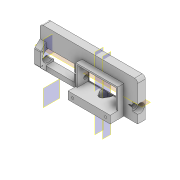
# Autodesk Inventor part: 10_Wellplate_base_v1
Saved by Autodesk Inventor 2022 (Build 260153000, 153)
## iProperties
Created: 2022-04-18
Part Number: 10_Wellplate_base_v1
Material: Generic
Document SubType Name: Modeling
Designer: Prakash Lab
Density: 1 g/cm^3
Appearance: Default
Author: Prakash Lab
Autodesk Inventor part; units mm, degrees
ref_plane "YZ Plane" through (0, 0, 0) normal (1, 0, 0) x (0, 1, 0)
ref_plane "XZ Plane" through (0, 0, 0) normal (0, 1, 0) x (-1, 0, 0)
ref_plane "XY Plane" through (0, 0, 0) normal (0, 0, 1) x (1, 0, 0)
sketch "Sketch1" plane through (0, 0, 0) normal (0, 0, 1) x (1, 0, 0)
  line L0 (63.9, -42.75) -> (-63.9, -42.75)
  line L1 (-63.9, -42.75) -> (-63.9, 42.75)
  line L2 (-63.9, 42.75) -> (63.9, 42.75)
  line L3 (63.9, 42.75) -> (63.9, -42.75)
  line L4 (63.9, -42.75) -> (-63.9, 42.75) construction
  line L5 (-63.9, -42.75) -> (63.9, 42.75) construction
  point P0 (0, 0)
  dimension "d0" = 127.8
  dimension "d1" = 85.5
  constraints: 12 end point, 2 midpoint, 2 parallel, 1 horizontal, 1 perpendicular
  measures "d0" distance of L0.start L0.end
  measures "d1" distance of L0.end L1.end
extrude "Extrusion1" add sketch "Sketch1" along normal blind 10
fillet "Fillet1" radius 4 4 edges at (63.9, 42.75, 5) (-63.9, 42.75, 5) (-63.9, -42.75, 5) (63.9, -42.75, 5)
sketch "Sketch2" plane through (0, 0, 10) normal (0, 0, 1) x (1, 0, 0)
  arc A0 (59.9, -42.75) -> (63.9, -38.75) centre (59.9, -38.75) ccw projected
  line L0 (63.9, -38.75) -> (63.9, 38.75) projected
  arc A1 (63.9, 38.75) -> (59.9, 42.75) centre (59.9, 38.75) ccw projected
  line L1 (59.9, 42.75) -> (-59.9, 42.75) projected
  arc A2 (-59.9, 42.75) -> (-63.9, 38.75) centre (-59.9, 38.75) ccw projected
  line L2 (-63.9, 38.75) -> (-63.9, -38.75) projected
  arc A3 (-63.9, -38.75) -> (-59.9, -42.75) centre (-59.9, -38.75) ccw projected
  line L3 (-59.9, -42.75) -> (59.9, -42.75) projected
  line L4 (43.9, 2.75) -> (-7.1, 2.75)
  line L5 (-7.1, 2.75) -> (-7.1, 27.75)
  line L6 (-7.1, 27.75) -> (43.9, 27.75)
  line L7 (43.9, 27.75) -> (43.9, 2.75)
  line L8 (43.9, 2.75) -> (-7.1, 27.75) construction
  line L9 (-7.1, 2.75) -> (43.9, 27.75) construction
  point P0 (0, 0)
  point P1 (18.4, 15.25)
  dimension "d5" = 51
  dimension "d6" = 25
  dimension "d7" = 20
  dimension "d8" = 15
  constraints: 12 end point, 2 midpoint, 2 parallel, 1 horizontal, 1 perpendicular
  measures "d5" distance of L5.end L6.end
  measures "d6" distance of L4.end L5.end
  measures "d7" distance between parallel lines of L0 L7
  measures "d8" distance between parallel lines of L6 L1
extrude "Extrusion2" cut sketch "Sketch2" against normal blind 6 contours L4 L5 L6 L7
sketch "Sketch3" plane through (0, 0, 4) normal (0, 0, 1) x (1, 0, 0)
  line L0 (-7.1, 27.75) -> (43.9, 27.75) projected
  line L1 (-7.1, 2.75) -> (-7.1, 27.75) projected
  line L2 (43.9, 2.75) -> (-7.1, 2.75) projected
  line L3 (43.9, 27.75) -> (43.9, 2.75) projected
  line L4 (42.4, 26.25) -> (-5.6, 26.25)
  line L5 (-5.6, 26.25) -> (-5.6, 4.25)
  line L6 (-5.6, 4.25) -> (42.4, 4.25)
  line L7 (42.4, 4.25) -> (42.4, 26.25)
  point P0 (0, 0)
  dimension "d11" = 1.5
  constraints: 8 end point, 3 other
  measures "d11" distance between parallel lines of L0 L4
extrude "Extrusion3" cut sketch "Sketch3" against normal through all contours L7 L6 L5 L4
ref_plane "Work Plane1" through (18.4, 2.75, 10) normal (-1, 0, 0) x (0, 0, 1)
ref_plane "Work Plane2" through (-7.1, 15.25, 10) normal (0, 1, 0) x (1, 0, 0)
chamfer "Chamfer1" distance 4 angle 45 4 edges at (18.4, 4.25, 0) (42.4, 15.25, 0) (18.4, 26.25, 0) (-5.6, 15.25, 0)
sketch "Sketch4" plane through (0, 0, 10) normal (0, 0, 1) x (1, 0, 0)
  line L0 (-7.1, 2.75) -> (-7.1, 27.75) projected
  line L1 (-7.1, 27.75) -> (43.9, 27.75) projected
  line L2 (43.9, 27.75) -> (43.9, 2.75) projected
  line L3 (43.9, 2.75) -> (-7.1, 2.75) projected
  arc A0 (59.9, -42.75) -> (63.9, -38.75) centre (59.9, -38.75) ccw projected
  line L4 (63.9, -38.75) -> (63.9, 38.75) projected
  arc A1 (63.9, 38.75) -> (59.9, 42.75) centre (59.9, 38.75) ccw projected
  line L5 (59.9, 42.75) -> (-59.9, 42.75) projected
  arc A2 (-59.9, 42.75) -> (-63.9, 38.75) centre (-59.9, 38.75) ccw projected
  line L6 (-63.9, 38.75) -> (-63.9, -38.75) projected
  arc A3 (-63.9, -38.75) -> (-59.9, -42.75) centre (-59.9, -38.75) ccw projected
  line L7 (-59.9, -42.75) -> (59.9, -42.75) projected
  line L8 (-7.1, 2.75) -> (43.9, 2.75)
  line L9 (43.9, 2.75) -> (43.9, -7.25)
  line L10 (43.9, -7.25) -> (-7.1, -7.25)
  line L11 (-7.1, -7.25) -> (-7.1, 2.75)
  line L12 (-7.1, 27.75) -> (43.9, 27.75) projected
  line L13 (-7.1, 27.75) -> (-9.1, 27.75)
  line L14 (-9.1, 27.75) -> (-9.1, -7.25)
  line L15 (-9.1, -7.25) -> (-7.1, -7.25)
  line L16 (-7.1, -7.25) -> (-7.1, 27.75)
  line L17 (43.9, 27.75) -> (45.9, 27.75)
  line L18 (45.9, 27.75) -> (45.9, -7.25)
  line L19 (45.9, -7.25) -> (43.9, -7.25)
  line L20 (43.9, -7.25) -> (43.9, 27.75)
  line L21 (45.9, 27.75) -> (-9.1, 27.75)
  line L22 (-9.1, 27.75) -> (-9.1, 29.75)
  line L23 (-9.1, 29.75) -> (45.9, 29.75)
  line L24 (45.9, 29.75) -> (45.9, 27.75)
  point P0 (0, 0)
  dimension "d17" = 10
  dimension "d52" = 2
  dimension "d53" = 2
  dimension "d54" = 2
  constraints: 32 end point, 8 parallel, 4 horizontal, 4 perpendicular, 2 point on line
  measures "d17" distance of L8.end L9.end
  measures "d52" distance of L15.end L14.end
  measures "d53" distance of L18.end L19.end
  measures "d54" distance of L21.end L22.end
extrude "Extrusion4" add sketch "Sketch4" along normal blind 8 contours L11 L15 L14 L13 L0 | L3 L9 L10 L11 | L13 L22 L23 L24 L17 L1 | L2 L17 L18 L19 L9
sketch "Sketch5" plane through (-7.1, 2.75, 4) normal (0, 1, 0) x (1, 0, 0)
  line L0 (22.0359, -8.925) -> (18.745, -3.225)
  line L1 (22.2091, 2.775) -> (28.7909, 2.775)
  line L2 (32.255, -3.225) -> (28.9641, -8.925)
  line L3 (53.5, 4) -> (-2.5, 4) projected
  circle A0 centre (25.5, -3.125) radius 0.95
  arc A1 (22.0359, -8.925) -> (28.9641, -8.925) centre (25.5, -6.925) ccw
  arc A2 (22.2091, 2.775) -> (18.745, -3.225) centre (22.2091, -1.225) ccw
  arc A3 (32.255, -3.225) -> (28.7909, 2.775) centre (28.7909, -1.225) ccw
  circle A4 centre (25.5, -3.125) radius 5.9
  circle A5 centre (25.5, -3.125) radius 6 projected
  point P0 (7.1, 4)
  point P1 (25.5, -14.925)
  point P2 (15.2809, 2.775)
  point P3 (35.7191, 2.775)
  dimension "d20" = 1.9
  dimension "d21" = 4
  dimension "d103" = 11.8
  constraints: 7 tangent, 6 end point, 6 point on circle, 6 point on line, 5 centre point, 3 coincident, 2 equal radius, 1 parallel, 7 other
  measures "d20" diameter of A0
  measures "d21" radius of A1
  measures "d103" diameter of A4
extrude "Extrusion5" cut sketch "Sketch5" against normal up to surface (10 mm away) contours L0 A5 L2 A1 | L0 A4 L2 A5 | L0 A5 L1 A4 | A4 | L0 A2 L1 A5 | L1 A5 L2 A4 | A5 L1 A3 L2 | A0
sketch "Sketch6" plane through (18.4, -7.25, 11.125) normal (0, -1, 0) x (1, 0, 0)
  circle A0 centre (0, -4) radius 7 projected
  circle A1 centre (0, -4) radius 10
  point P0 (-18.4, -11.125)
  dimension "d27" = 20
  constraints: 1 centre point, 1 coincident
  measures "d27" diameter of A1
extrude "Extrusion6" cut sketch "Sketch6" along normal blind 18 contours A0 | A1
ref_plane "Work Plane3" through (8.4, 2.75, 10) normal (-1, 0, 0) x (0, 0, 1)
sketch "Sketch12" plane through (63.9, -38.75, 0) normal (1, 0, 0) x (0, 0, -1)
  circle A0 centre (-7.125, 48) radius 4.2 construction
  circle A1 centre (-7.125, 48) radius 3.5
  point P0 (0, 38.75)
  dimension "d100" = 7
  constraints: 1 centre point
  measures "d100" diameter of A1
extrude "Extrusion12" cut sketch "Sketch12" against normal blind 30 draft -3
sketch "Sketch13" plane through (63.9, -38.75, 0) normal (1, 0, 0) x (0, 0, -1)
  arc A0 (-10, 44.9382) -> (-10, 51.0618) centre (-7.125, 48) ccw projected
  circle A1 centre (-7.125, 48) radius 6
  point P0 (0, 38.75)
  dimension "d63" = 12
  constraints: 1 centre point, 1 coincident
  measures "d63" diameter of A1
extrude "Extrusion13" cut sketch "Sketch13" against normal blind 7
mirror "Mirror1" about plane through (18.4, 2.75, 10) normal (-1, 0, 0) of "Extrusion12", "Extrusion13"
ref_plane "Work Plane4" through (-47.9, 27.75, 11) normal (-1, 0, 0) x (0, 0, 1)
ref_plane "Work Plane5" through (-39.7, 19.25, 21) normal (0, 0, 1) x (1, 0, 0)
sketch "Sketch22" plane through (0, 0, 18) normal (0, 0, 1) x (1, 0, 0)
  line L0 (-7.1, 2.75) -> (-7.1, 27.75) projected
  line L1 (-7.1, 27.75) -> (43.9, 27.75) projected
  line L2 (43.9, 27.75) -> (43.9, 2.75) projected
  line L3 (43.9, 2.75) -> (-7.1, 2.75) projected
  line L4 (-9.1, -7.25) -> (45.9, -7.25) projected
  line L5 (45.9, -7.25) -> (45.9, 29.75) projected
  line L6 (45.9, 29.75) -> (-9.1, 29.75) projected
  line L7 (-9.1, 29.75) -> (-9.1, -7.25) projected
  line L8 (45.9, -7.25) -> (45.9, 29.75) projected
  line L9 (45.9, 2.75) -> (-9.1, 2.75)
  point P0 (0, 0)
  point P1 (43.9, 2.75)
  constraints: 2 end point, 2 point on line, 1 perpendicular
extrude "Extrusion21" add sketch "Sketch22" along normal blind 10 contours L3 L9 L5 L4 L7
sketch "Sketch23" plane through (0, 0, 28) normal (0, 0, 1) x (1, 0, 0)
  line L0 (45.9, -7.25) -> (45.9, 2.75) projected
  line L1 (45.9, 2.75) -> (-9.1, 2.75) projected
  line L2 (-9.1, 2.75) -> (-9.1, -7.25) projected
  line L3 (-9.1, -7.25) -> (45.9, -7.25) projected
  circle A0 centre (39.9, -2.25) radius 1.4
  circle A1 centre (-3.1, -2.25) radius 1.4
  point P0 (0, 0)
  dimension "d105" = 2.8
  dimension "d106" = 2.8
  dimension "d107" = 6
  dimension "d108" = 6
  constraints: 2 centre point
  measures "d105" diameter of A0
  measures "d106" diameter of A1
  measures "d107" distance from line of A0.centre L0
  measures "d108" distance from line of A1.centre L2
extrude "Extrusion22" cut sketch "Sketch23" against normal through all contours A0 | A1
ref_plane "Arbeitsebene7" through (-58.9, -38.75, 0) normal (-1, 0, 0) x (0, 0, 1)
sketch "Skizze28" plane through (-58.9, -38.75, 0) normal (-1, 0, 0) x (0, 0, 1)
  line L0 (17.125, 56.5) -> (17.125, 39.5) projected
  arc A0 (17.125, 56.5) -> (15.625, 58) centre (15.625, 56.5) ccw projected
  line L1 (-1.375, 58) -> (15.625, 58) projected
  arc A1 (-1.375, 58) -> (-2.875, 56.5) centre (-1.375, 56.5) ccw projected
  line L2 (-2.875, 39.5) -> (-2.875, 56.5) projected
  arc A2 (-2.875, 39.5) -> (-1.375, 38) centre (-1.375, 39.5) ccw projected
  line L3 (15.625, 38) -> (-1.375, 38) projected
  arc A3 (15.625, 38) -> (17.125, 39.5) centre (15.625, 39.5) ccw projected
  circle A4 centre (15.125, 56) radius 0.7835 projected
  circle A5 centre (15.125, 40) radius 0.7835 projected
  circle A6 centre (-0.875, 56) radius 0.7835 projected
  circle A7 centre (-0.875, 40) radius 0.7835 projected
  circle A8 centre (7.125, 48) radius 7.5 projected
  arc A9 (17.625, 56.5) -> (15.625, 58.5) centre (15.625, 56.5) ccw
  line L4 (17.625, 56.5) -> (17.625, 39.5)
  arc A10 (15.625, 37.5) -> (17.625, 39.5) centre (15.625, 39.5) ccw
  line L5 (15.625, 37.5) -> (-1.375, 37.5)
  arc A11 (-3.375, 39.5) -> (-1.375, 37.5) centre (-1.375, 39.5) ccw
  line L6 (-3.375, 39.5) -> (-3.375, 56.5)
  arc A12 (-1.375, 58.5) -> (-3.375, 56.5) centre (-1.375, 56.5) ccw
  line L7 (-1.375, 58.5) -> (15.625, 58.5)
  point P0 (0, 38.75)
  dimension "d142" = 0.5
  constraints: 8 end point, 8 point on circle, 4 centre point, 7 other
  measures "d142" distance between parallel lines of L1 L7
extrude "Extrusion27" cut sketch "Skizze28" against normal blind 40 contours L0 A3 L3 A2 L2 A1 L1 A0 | A4 | A5 | A6 | A7 | A8 | L4 A10 L5 A11 L6 A12 L7 A9
sketch "Skizze29" plane through (-63.9, -38.75, 0) normal (-1, 0, 0) x (0, 0, 1)
  line L0 (17.125, 56.5) -> (17.125, 39.5) projected
  arc A0 (17.125, 56.5) -> (15.625, 58) centre (15.625, 56.5) ccw projected
  line L1 (-1.375, 58) -> (15.625, 58) projected
  arc A1 (-1.375, 58) -> (-2.875, 56.5) centre (-1.375, 56.5) ccw projected
  line L2 (-2.875, 39.5) -> (-2.875, 56.5) projected
  arc A2 (-2.875, 39.5) -> (-1.375, 38) centre (-1.375, 39.5) ccw projected
  line L3 (15.625, 38) -> (-1.375, 38) projected
  arc A3 (15.625, 38) -> (17.125, 39.5) centre (15.625, 39.5) ccw projected
  circle A4 centre (15.125, 56) radius 0.7835 projected
  circle A5 centre (15.125, 40) radius 0.7835 projected
  circle A6 centre (-0.875, 56) radius 0.7835 projected
  circle A7 centre (-0.875, 40) radius 0.7835 projected
  circle A8 centre (7.125, 48) radius 7.5 projected
  line L4 (0, 77.5) -> (0, 0) projected
  line L5 (10, 77.5) -> (10, 0) projected
  line L6 (10, 0) -> (10, 42.7337) projected
  line L7 (10, 31.7537) -> (16.6857, 38.4393)
  line L8 (16.6857, 57.5607) -> (10, 64.2463)
  line L9 (10, 68.5) -> (10, 31.5) projected
  point P0 (0, 38.75)
  point P1 (0, 58)
  point P2 (0, 38)
  point P3 (10, 11.9077)
  point P4 (10, 38)
  point P5 (10, 58)
  point P6 (10, 10.3787)
  dimension "d151" = 45
  dimension "d152" = 45
  constraints: 4 end point, 2 point on circle, 2 point on line
  measures "d151" angle of L1 L8
  measures "d152" angle of L3 L7
extrude "Extrusion28" add sketch "Skizze29" against normal blind 8 contours L0 A3 L3 L5 A8 L1 A0 | A0 L1 L5 L8 | L7 L5 L3 A3 | L5 A8 L4 L1 | L3 L4 A8 L5 | L5 A8 L4 | A8 L5
sketch "Skizze30" plane through (-55.9, -38.75, 0) normal (1, 0, 0) x (0, 0, -1)
  circle A0 centre (-7.125, 48) radius 7.3 projected
  circle A1 centre (-7.125, 48) radius 7.8
  point P0 (0, 38.75)
  dimension "d147" = 0.5
  constraints: 1 centre point
  measures "d147" radial gap between concentric circles of A0 A1
extrude "Extrusion29" cut sketch "Skizze30" against normal up to surface (8 mm away) contours A0 | A1
fillet "Rundung6" radius 2 2 edges at (-59.9, 6.076, 0) (-59.9, 12.424, 0)
sketch "Skizze32" plane through (-63.9, -38.75, 0) normal (-1, 0, 0) x (0, 0, 1)
  circle A0 centre (5.1474, 11) radius 6.7945 projected
  point P0 (0, 38.75)
ref_plane "Arbeitsebene8" through (-41.36, -34.2905, -1.3931) normal (1, 0, 0) x (0, 1, 0)
extrude "Extrusion30" cut sketch "Skizze32" against normal up to surface (22.54 mm away)
sketch "Skizze33" plane through (-41.36, -32.5058, 10) normal (-1, 0, 0) x (0, 0, 1)
  arc A0 (-5.8686, 8.6246) -> (-3.8366, 8.6246) centre (-4.8526, 4.7558) ccw projected
  circle A1 centre (-4.8526, 4.7558) radius 3.5
  line L0 (-4.8526, 8.2558) -> (5.2065, 8.2558)
  line L1 (5.2065, 8.2558) -> (5.2065, 1.2558)
  line L2 (5.2065, 1.2558) -> (-4.8526, 1.2558)
  line L3 (-4.8526, 1.2558) -> (-4.8526, 8.2558)
  point P0 (-10, 32.5058)
  point P1 (-4.8526, 1.2558)
  dimension "d155" = 7
  constraints: 8 end point, 2 parallel, 1 coincident, 1 horizontal, 1 perpendicular, 3 other
extrude "Extrusion31" cut sketch "Skizze33" against normal blind 3
sketch "Skizze34" plane through (-38.36, -32.5058, 10) normal (-1, 0, 0) x (0, 0, 1)
  circle A0 centre (-4.8526, 4.7558) radius 6.5405 projected
  circle A1 centre (-4.8526, 4.7558) radius 8.5
  line L0 (-4.8526, 13.2558) -> (8.37, 13.2558)
  line L1 (8.37, 13.2558) -> (8.37, -3.7442)
  line L2 (8.37, -3.7442) -> (-4.8526, -3.7442)
  line L3 (-4.8526, -3.7442) -> (-4.8526, 13.2558)
  point P0 (-10, 32.5058)
  point P1 (-4.8526, -3.7442)
  dimension "d160" = 17
  constraints: 8 end point, 2 parallel, 1 coincident, 1 horizontal, 1 perpendicular, 3 other
extrude "Extrusion32" cut sketch "Skizze34" against normal blind 30
sketch "Skizze35" plane through (-38.36, -32.5058, 10) normal (1, 0, 0) x (0, 0, -1)
  line L0 (10, 11.52) -> (10, -2.0084) projected
  arc A0 (10, 11.52) -> (4.8526, 13.2558) centre (4.8526, 4.7558) ccw projected
  line L1 (0, 13.2558) -> (4.8526, 13.2558) projected
  line L2 (0, 8.2558) -> (0, 13.2558) projected
  line L3 (4.8526, 8.2558) -> (0, 8.2558) projected
  arc A1 (4.8526, 1.2558) -> (4.8526, 8.2558) centre (4.8526, 4.7558) ccw projected
  line L4 (0, 1.2558) -> (4.8526, 1.2558) projected
  line L5 (0, -3.7442) -> (0, 1.2558) projected
  line L6 (4.8526, -3.7442) -> (0, -3.7442) projected
  arc A2 (4.8526, -3.7442) -> (10, -2.0084) centre (4.8526, 4.7558) ccw projected
  circle A3 centre (4.8526, 4.7558) radius 6 projected
  line L7 (4.8526, 10.7558) -> (0, 10.7558)
  line L8 (4.8526, -1.2442) -> (0, -1.2442)
  line L9 (0, -3.7442) -> (0, 1.2558) projected
  point P0 (10, 32.5058)
  point P1 (10, 1.6729)
  point P2 (0, -1.2442)
  point P3 (10, 7.8387)
  constraints: 4 end point, 2 midpoint, 2 point on circle
extrude "Extrusion33" add sketch "Skizze35" along normal blind 15 contours L0 A3 L7 L2 L1 A0 | L0 A2 L6 L5 L8 A3
sketch "Skizze36" plane through (0, 0, 10) normal (0, 0, 1) x (1, 0, 0)
  line L0 (20.65, -24.75) -> (15.25, -24.75) projected
  line L1 (15.25, -24.75) -> (15.25, -31.55) projected
  line L2 (20.65, -31.55) -> (15.25, -31.55) projected
  line L3 (20.65, -31.55) -> (20.65, -24.75) projected
  line L4 (14.75, -32.05) -> (14.75, -24.25)
  line L5 (14.75, -24.25) -> (21.15, -24.25)
  line L6 (21.15, -24.25) -> (21.15, -32.05)
  line L7 (21.15, -32.05) -> (14.75, -32.05)
  point P0 (0, 0)
  dimension "d163" = 0.5
  constraints: 8 end point, 3 other
  measures "d163" distance between parallel lines of L1 L4
ref_plane "Arbeitsebene9" through (15.25, -31.55, 0.625) normal (0, 0, -1) x (0, 1, 0)
extrude "Extrusion34" cut sketch "Skizze36" against normal up to surface (9.375 mm away) contours L3 L2 L1 L0 | L4 L5 L6 L7
sketch "Skizze37" plane through (-8.36, -32.5058, 10) normal (-1, 0, 0) x (0, 0, 1)
  circle A0 centre (-4.8526, 4.7558) radius 6.5405 projected
  circle A1 centre (-4.8526, 4.7558) radius 4
  line L0 (-4.8526, 0.7558) -> (5.4732, 0.7558)
  line L1 (5.4732, 0.7558) -> (5.4732, 8.7558)
  line L2 (5.4732, 8.7558) -> (-4.8526, 8.7558)
  line L3 (-4.8526, 8.7558) -> (-4.8526, 0.7558)
  point P0 (-10, 32.5058)
  point P1 (-4.8526, 8.7558)
  dimension "d166" = 8
  constraints: 8 end point, 2 parallel, 1 coincident, 1 horizontal, 1 perpendicular, 3 other
extrude "Extrusion35" cut sketch "Skizze37" against normal up to surface (23.11 mm away) contours A0 L0 A1 L2 | A0 L2 L1 L0 | L3 A1 | A1 L3 picked at (0.7888, 4.2814)
sketch "Skizze38" plane through (0, 0, 10) normal (0, 0, 1) x (1, 0, 0)
  line L0 (-8.36, -23.75) -> (8.8222, -23.75) projected
  line L1 (8.8222, -23.75) -> (8.8222, -7.25) projected
  line L2 (8.8222, -7.25) -> (-9.1, -7.25) projected
  line L3 (-9.1, -7.25) -> (-9.1, 29.75) projected
  line L4 (-9.1, 29.75) -> (45.9, 29.75) projected
  line L5 (45.9, 29.75) -> (45.9, -7.25) projected
  line L6 (45.9, -7.25) -> (27.9778, -7.25) projected
  line L7 (27.9778, -7.25) -> (27.9778, -25.25) projected
  line L8 (27.9778, -25.25) -> (21.15, -25.25) projected
  line L9 (21.15, -25.25) -> (21.15, -32.05) projected
  line L10 (21.15, -32.05) -> (14.75, -32.05) projected
  line L11 (14.75, -32.05) -> (14.75, -31.75) projected
  line L12 (14.75, -31.75) -> (-8.36, -31.75) projected
  line L13 (-8.36, -31.75) -> (-8.36, -36.25) projected
  line L14 (-8.36, -36.25) -> (-23.36, -36.25) projected
  line L15 (-23.36, -33.75) -> (-23.36, -36.25) projected
  line L16 (-38.36, -33.75) -> (-23.36, -33.75) projected
  line L17 (-38.36, -33.75) -> (-38.36, -31.25) projected
  line L18 (-38.36, -31.25) -> (-41.36, -31.25) projected
  line L19 (-41.36, -31.25) -> (-41.36, -32.5058) projected
  line L20 (-41.36, -32.5058) -> (-63.9, -32.5058) projected
  line L21 (-63.9, -32.5058) -> (-63.9, -38.75) projected
  arc A0 (-63.9, -38.75) -> (-59.9, -42.75) centre (-59.9, -38.75) ccw projected
  line L22 (-59.9, -42.75) -> (59.9, -42.75) projected
  arc A1 (59.9, -42.75) -> (63.9, -38.75) centre (59.9, -38.75) ccw projected
  line L23 (63.9, -38.75) -> (63.9, 3.9837) projected
  line L24 (63.9, 3.9837) -> (56.9, 3.9837) projected
  line L25 (56.9, 3.9837) -> (56.9, 8.0046) projected
  line L26 (56.9, 10.4954) -> (56.9, 14.5163) projected
  line L27 (56.9, 14.5163) -> (63.9, 14.5163) projected
  line L28 (63.9, 14.5163) -> (63.9, 38.75) projected
  arc A2 (63.9, 38.75) -> (59.9, 42.75) centre (59.9, 38.75) ccw projected
  line L29 (59.9, 42.75) -> (-59.9, 42.75) projected
  arc A3 (-59.9, 42.75) -> (-63.9, 38.75) centre (-59.9, 38.75) ccw projected
  line L30 (-63.9, 38.75) -> (-63.9, 25.4963) projected
  line L31 (-63.9, 25.4963) -> (-55.9, 25.4963) projected
  line L32 (-55.9, 25.4963) -> (-55.9, 19.75) projected
  line L33 (-55.9, 19.75) -> (-18.9, 19.75) projected
  line L34 (-18.9, 19.75) -> (-18.9, 10.3274) projected
  line L35 (-18.9, 8.1726) -> (-18.9, -1.25) projected
  line L36 (-18.9, -1.25) -> (-55.9, -1.25) projected
  line L37 (-55.9, -1.25) -> (-55.9, -6.9963) projected
  line L38 (-55.9, -6.9963) -> (-63.9, -6.9963) projected
  line L39 (-63.9, -6.9963) -> (-63.9, -22.9942) projected
  line L40 (-63.9, -22.9942) -> (-41.36, -22.9942) projected
  line L41 (-41.36, -22.9942) -> (-41.36, -24.25) projected
  line L42 (-41.36, -24.25) -> (-38.36, -24.25) projected
  line L43 (-38.36, -24.25) -> (-38.36, -21.75) projected
  line L44 (-38.36, -21.75) -> (-23.36, -21.75) projected
  line L45 (-23.36, -19.25) -> (-23.36, -21.75) projected
  line L46 (-23.36, -19.25) -> (-8.36, -19.25) projected
  line L47 (-8.36, -19.25) -> (-8.36, -23.75) projected
  point P0 (0, 0)
  point P1 (-42.2276, -36.25)
  point P2 (-42.2276, -19.25)
  point P3 (-27.8589, -14.9953)
  point P4 (-27.8589, -39.949)
  point P5 (17.95, -36.25)
  point P6 (27.4914, -28.65)
  point P7 (5.4922, -12.0867)
  point P8 (32.285, -12.0867)
  constraints: 2 vertical alignment
hole "Bohrung2" at (-42.2276, -36.25, 10) at (-42.2276, -19.25, 10) at (-27.8589, -14.9953, 10) at (-27.8589, -39.949, 10) at (17.95, -36.25, 10) at (27.4914, -28.65, 10) at (5.4922, -12.0867, 10) at (32.285, -12.0867, 10) direction (0, 0, -1) diameter 2.8 end through all
sketch "Skizze39" plane through (0, 0, 10) normal (0, 0, 1) x (1, 0, 0)
  circle A0 centre (5.4922, -12.0867) radius 1.4 projected
  circle A1 centre (17.95, -36.25) radius 1.4 projected
  circle A2 centre (-27.8589, -14.9953) radius 1.4 projected
  circle A3 centre (-42.2276, -36.25) radius 1.4 projected
  circle A4 centre (-42.2276, -19.25) radius 1.4 projected
  circle A5 centre (-27.8589, -39.949) radius 1.4 projected
  circle A6 centre (27.4914, -28.65) radius 1.4 projected
  circle A7 centre (32.285, -12.0867) radius 1.4 projected
  line L0 (-8.36, -23.75) -> (8.8222, -23.75) projected
  line L1 (8.8222, -23.75) -> (8.8222, -7.25) projected
  line L2 (8.8222, -7.25) -> (-9.1, -7.25) projected
  line L3 (-9.1, -7.25) -> (-9.1, 29.75) projected
  line L4 (-9.1, 29.75) -> (45.9, 29.75) projected
  line L5 (45.9, 29.75) -> (45.9, -7.25) projected
  line L6 (45.9, -7.25) -> (27.9778, -7.25) projected
  line L7 (27.9778, -7.25) -> (27.9778, -25.25) projected
  line L8 (27.9778, -25.25) -> (21.15, -25.25) projected
  line L9 (21.15, -25.25) -> (21.15, -32.05) projected
  line L10 (21.15, -32.05) -> (14.75, -32.05) projected
  line L11 (14.75, -32.05) -> (14.75, -31.75) projected
  line L12 (14.75, -31.75) -> (-8.36, -31.75) projected
  line L13 (-8.36, -31.75) -> (-8.36, -36.25) projected
  line L14 (-8.36, -36.25) -> (-23.36, -36.25) projected
  line L15 (-23.36, -33.75) -> (-23.36, -36.25) projected
  line L16 (-38.36, -33.75) -> (-23.36, -33.75) projected
  line L17 (-38.36, -33.75) -> (-38.36, -31.25) projected
  line L18 (-38.36, -31.25) -> (-41.36, -31.25) projected
  line L19 (-41.36, -31.25) -> (-41.36, -32.5058) projected
  line L20 (-41.36, -32.5058) -> (-63.9, -32.5058) projected
  line L21 (-63.9, -32.5058) -> (-63.9, -38.75) projected
  arc A8 (-63.9, -38.75) -> (-59.9, -42.75) centre (-59.9, -38.75) ccw projected
  line L22 (-59.9, -42.75) -> (59.9, -42.75) projected
  arc A9 (59.9, -42.75) -> (63.9, -38.75) centre (59.9, -38.75) ccw projected
  line L23 (63.9, -38.75) -> (63.9, 3.9837) projected
  line L24 (63.9, 3.9837) -> (56.9, 3.9837) projected
  line L25 (56.9, 3.9837) -> (56.9, 8.0046) projected
  line L26 (56.9, 10.4954) -> (56.9, 14.5163) projected
  line L27 (56.9, 14.5163) -> (63.9, 14.5163) projected
  line L28 (63.9, 14.5163) -> (63.9, 38.75) projected
  arc A10 (63.9, 38.75) -> (59.9, 42.75) centre (59.9, 38.75) ccw projected
  line L29 (59.9, 42.75) -> (-59.9, 42.75) projected
  arc A11 (-59.9, 42.75) -> (-63.9, 38.75) centre (-59.9, 38.75) ccw projected
  line L30 (-63.9, 38.75) -> (-63.9, 25.4963) projected
  line L31 (-63.9, 25.4963) -> (-55.9, 25.4963) projected
  line L32 (-55.9, 25.4963) -> (-55.9, 19.75) projected
  line L33 (-55.9, 19.75) -> (-18.9, 19.75) projected
  line L34 (-18.9, 19.75) -> (-18.9, 10.3274) projected
  line L35 (-18.9, 8.1726) -> (-18.9, -1.25) projected
  line L36 (-18.9, -1.25) -> (-55.9, -1.25) projected
  line L37 (-55.9, -1.25) -> (-55.9, -6.9963) projected
  line L38 (-55.9, -6.9963) -> (-63.9, -6.9963) projected
  line L39 (-63.9, -6.9963) -> (-63.9, -22.9942) projected
  line L40 (-63.9, -22.9942) -> (-41.36, -22.9942) projected
  line L41 (-41.36, -22.9942) -> (-41.36, -24.25) projected
  line L42 (-41.36, -24.25) -> (-38.36, -24.25) projected
  line L43 (-38.36, -24.25) -> (-38.36, -21.75) projected
  line L44 (-38.36, -21.75) -> (-23.36, -21.75) projected
  line L45 (-23.36, -19.25) -> (-23.36, -21.75) projected
  line L46 (-23.36, -19.25) -> (-8.36, -19.25) projected
  line L47 (-8.36, -19.25) -> (-8.36, -23.75) projected
  line L48 (63.9, -38.75) -> (63.9, 38.75) projected
  line L49 (63.9, -7.25) -> (-65.3546, -7.25)
  line L50 (-65.3546, -7.25) -> (-65.3546, -46.5164)
  line L51 (-65.3546, -46.5164) -> (63.9, -46.5164)
  line L52 (63.9, -46.5164) -> (63.9, -7.25)
  point P0 (0, 0)
  point P1 (45.9, -7.25)
  constraints: 8 end point, 2 parallel, 2 vertical alignment, 1 horizontal, 1 perpendicular, 1 point on line
extrude "Extrusion36" cut sketch "Skizze39" along normal through all both and the other way through all contours A0 | A1 | A2 | A3 | A4 | A5 | A6 | A7 | L47 L46 L45 L44 L43 L42 L41 L40 L39 L49 L2 L1 L0 | L0 L1 L49 L7 L8 L9 L10 L11 L12 L13 L14 L15 L16 L17 L18 L19 L20 L21 A8 L22 A9 L52 L51 L50 L39 L40 L41 L42 L43 L44 L45 L46 L47 | L6 L49 L23 A9 L22 A8 L21 L20 L19 L18 L17 L16 L15 L14 L13 L12 L11 L10 L9 L8 L7
body "Solid1"
